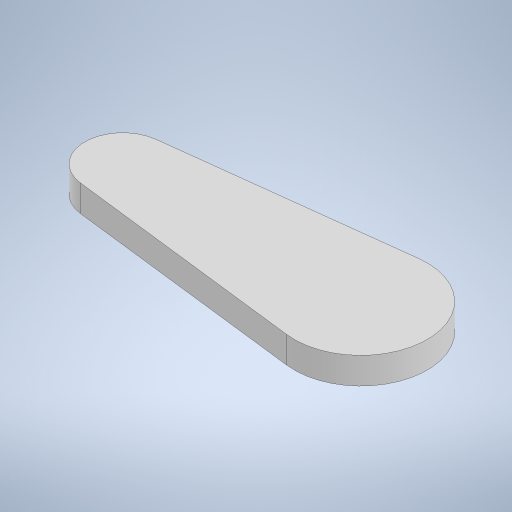
# Autodesk Inventor part: Arm
Saved by Autodesk Inventor 2023.2 (Build 272271000, 271)
## iProperties
Created: 2022-12-06
Part Number: Arm
Material: Generic
Document SubType Name: Modeling
Designer: Team 4026
Density: 1 g/cm^3
Appearance: Default
Author: Team 4026
Autodesk Inventor part; units mm, degrees
ref_plane "YZ Plane" through (0, 0, 0) normal (1, 0, 0) x (0, 1, 0)
ref_plane "XZ Plane" through (0, 0, 0) normal (0, 1, 0) x (-1, 0, 0)
ref_plane "XY Plane" through (0, 0, 0) normal (0, 0, 1) x (1, 0, 0)
sketch "Sketch4" plane through (0, 0, 0) normal (0, 1, 0) x (-1, 0, 0)
  circle A0 centre (30.8963, 0) radius 12.7 construction
  circle A1 centre (-45.3037, 0) radius 19.05 construction
  line L0 (-45.3037, 0) -> (30.8963, 0) construction
  line L1 (24.2814, 10.8413) -> (-43.0353, 18.9145) construction
  line L2 (24.2814, -10.8413) -> (-43.0353, -18.9145) construction
  line L3 (24.2814, 10.8413) -> (-43.0353, 18.9145)
  line L4 (24.2814, -10.8413) -> (-43.0353, -18.9145)
  arc A2 (24.2814, -10.8413) -> (24.2814, 10.8413) centre (22.9813, 0) ccw
  arc A3 (-43.0353, 18.9145) -> (-43.0353, -18.9145) centre (-45.3037, 0) ccw
  point P0 (0, 0)
  dimension "d4" = 25.4
  dimension "d5" = 38.1
  dimension "d6" = 76.2
  constraints: 10 end point, 8 point on circle, 7 tangent, 4 centre point, 1 horizontal
  measures "d4" diameter of A0
  measures "d5" diameter of A1
  measures "d6" distance of L0.start L0.end
extrude "Extrusion1" add sketch "Sketch4" along normal blind 7.62
body "Solid1"
